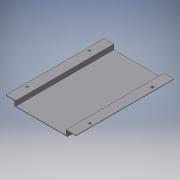
# Autodesk Inventor part: PCB-Mount
Saved by Autodesk Inventor 2016 SP2 (Build 200236200, 236)
## iProperties
Created: 2018-08-07
Part Number: PCB-Mount
Material: Generisch
Document SubType Name: Modeling
Designer: Nils
Density: 1 g/cm^3
Appearance: Vorgabe
Author: Nils
Autodesk Inventor part; units mm, degrees
ref_plane "YZ Plane" through (0, 0, 0) normal (1, 0, 0) x (0, 1, 0)
ref_plane "XZ Plane" through (0, 0, 0) normal (0, 1, 0) x (-1, 0, 0)
ref_plane "XY Plane" through (0, 0, 0) normal (0, 0, 1) x (1, 0, 0)
sketch "Skizze1" plane through (0, 0, 0) normal (0, 0, 1) x (1, 0, 0)
  line L0 (-90, 421.0534) -> (-90, 451.3884) construction
  line L1 (-90, 311.0534) -> (10, 311.0534)
  line L2 (10, 311.0534) -> (10, 451.0534)
  line L3 (10, 451.0534) -> (-90, 451.0534)
  line L4 (-90, 451.0534) -> (-90, 311.0534)
  circle A0 centre (5, 336.0534) radius 1.55 projected
  circle A1 centre (-85, 425.3034) radius 1.75 projected
  line L5 (10, 304.3034) -> (10, 341.0534) projected
  circle A2 centre (-85, 336.0534) radius 1.55 projected
  circle A3 centre (5, 425.3034) radius 1.75 projected
  line L6 (-90, 304.3034) -> (-90, 341.0534) construction
  point P0 (0, 0)
  dimension "d14" = 25.75
  dimension "d15" = 25
  constraints: 10 end point, 2 collinear, 2 parallel, 1 horizontal, 1 perpendicular
  measures "d14" distance from line of L3 A1.centre
  measures "d15" distance from line of L1 A2.centre
extrude "Extrusion1" add sketch "Skizze1" along normal blind 0.6
sketch "Skizze2" plane through (0, 0, 0) normal (0, 0, -1) x (-1, 0, 0)
  line L0 (90, 311.0534) -> (-10, 311.0534) projected
  line L1 (-10, 451.0534) -> (90, 451.0534) projected
  line L2 (2, 311.0534) -> (78, 311.0534)
  line L3 (78, 311.0534) -> (78, 451.0534)
  line L4 (78, 451.0534) -> (2, 451.0534)
  line L5 (2, 451.0534) -> (2, 311.0534)
  line L6 (-10, 311.0534) -> (-10, 451.0534) projected
  line L7 (90, 451.0534) -> (90, 311.0534) projected
  line L8 (78, 451.0534) -> (2, 451.0534)
  line L9 (2, 451.0534) -> (2, 311.0534)
  line L10 (2, 311.0534) -> (78, 311.0534)
  line L11 (78, 311.0534) -> (78, 451.0534)
  point P0 (0, 0)
  dimension "d4" = 12
  dimension "d5" = 12
  constraints: 16 end point, 4 parallel, 2 horizontal, 2 perpendicular, 2 point on line
  measures "d4" distance between parallel lines of L6 L5
  measures "d5" distance between parallel lines of L7 L3
extrude "Extrusion3" add sketch "Skizze2" along normal blind 7 contours L0 L5 L1 L3
sketch "Skizze3" plane through (0, 0, 0.6) normal (0, 0, 1) x (1, 0, 0)
  line L0 (-2, 311.0534) -> (-78, 311.0534) construction
  line L1 (-78, 311.0534) -> (-78, 451.0534) construction
  line L2 (-78, 451.0534) -> (-2, 451.0534) construction
  line L3 (-2, 451.0534) -> (-2, 311.0534) construction
  line L4 (-90, 311.0534) -> (10, 311.0534) projected
  line L5 (-78, 451.0534) -> (-2, 451.0534) projected
  line L6 (-4, 311.0534) -> (-76, 311.0534)
  line L7 (-76, 311.0534) -> (-76, 451.0534)
  line L8 (-76, 451.0534) -> (-4, 451.0534)
  line L9 (-4, 451.0534) -> (-4, 311.0534)
  point P0 (0, 0)
  dimension "d10" = 2
  dimension "d11" = 2
  constraints: 8 end point, 2 parallel, 2 point on line, 1 horizontal, 1 perpendicular
  measures "d10" distance between parallel lines of L1 L7
  measures "d11" distance between parallel lines of L3 L9
extrude "Extrusion4" cut sketch "Skizze3" against normal blind 7
